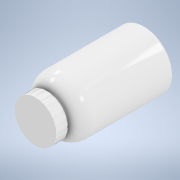
# Autodesk Inventor part: Healing-Iteam-Pills
Saved by Autodesk Inventor 2020 (Build 240168000, 168)
## iProperties
Created: 2019-09-13
Part Number: Healing-Iteam-Pills
Material: Generic
Document SubType Name: Modeling
Designer: vifly_01
Density: 1 g/cm^3
Appearance: Default
Author: vifly_01
Autodesk Inventor part; units mm, degrees
ref_plane "YZ Plane" through (0, 0, 0) normal (1, 0, 0) x (0, 1, 0)
ref_plane "XZ Plane" through (0, 0, 0) normal (0, 1, 0) x (-1, 0, 0)
ref_plane "XY Plane" through (0, 0, 0) normal (0, 0, 1) x (1, 0, 0)
sketch "Sketch1" plane through (0, 0, 0) normal (0, 0, 1) x (1, 0, 0)
  circle A0 centre (0, 0) radius 7.5
  dimension "d0" = 15
  constraints: 1 centre point, 1 coincident
  measures "d0" diameter of A0
extrude "Extrusion1" add sketch "Sketch1" along normal blind 20
sketch "Sketch3" plane through (0, 0, 0) normal (1, 0, 0) x (0, 1, 0)
  line L0 (7.5, 20) -> (-7.5, 20) projected
  arc A0 (7.5, 20) -> (4.75, 25) centre (2.4104, 20.457) ccw
  line L1 (4.75, 25) -> (4.75, 20)
  line L2 (7.5, 20) -> (4.75, 20)
  line L3 (0, -5.128) -> (0, 30.7682) projected
  point P0 (0, 0)
  dimension "d3" = 5
  dimension "d4" = 2.75
  constraints: 4 end point, 2 point on circle, 1 centre point, 1 collinear, 1 perpendicular, 1 point on line
  measures "d3" distance from line of L0 L1.start
  measures "d4" horizontal distance of L0.start L1.start
revolve "Revolution1" add sketch "Sketch3" angle 360 about axis through (0, 0, -10) along (0, 0, 1)
sketch "Sketch4" plane through (0, 0, 20) normal (0, 0, 1) x (1, 0, 0)
  circle A0 centre (0, 0) radius 4.75
  constraints: 1 centre point, 1 coincident
extrude "Extrusion2" add sketch "Sketch4" along normal blind 5.75
sketch "Sketch5" plane through (0, 0, 25.75) normal (0, 0, 1) x (1, 0, 0)
  circle A0 centre (0, 0) radius 5.5
  dimension "d8" = 11
  constraints: 1 centre point, 1 coincident
  measures "d8" diameter of A0
extrude "Extrusion3" add sketch "Sketch5" along normal blind 3
sketch "Sketch6" plane through (0, 0, 28.75) normal (0, 0, 1) x (1, 0, 0)
  arc A0 (-5.4899, 0.3337) -> (-5.5, 0) centre (0, 0) ccw
  circle A1 centre (0, 0) radius 5.5 projected
  arc A2 (-5.4398, 0.3337) -> (-5.45, 0) centre (0, 0) ccw
  line L0 (-5.4398, 0.3337) -> (-5.4899, 0.3337)
  line L1 (-5.45, 0) -> (-5.5, 0)
  line L2 (-5.6591, 0) -> (-5.2331, 0)
  arc A3 (-5.5, 0) -> (-5.4899, -0.3337) centre (0, 0) ccw
  arc A4 (-5.45, 0) -> (-5.4398, -0.3337) centre (0, 0) ccw
  line L3 (-5.4398, -0.3337) -> (-5.4899, -0.3337)
  point P0 (-5.4899, -0.3337)
  dimension "d14" = 0.05
  constraints: 10 point on circle, 8 end point, 4 centre point, 2 horizontal, 2 symmetric about line, 1 coincident, 1 parallel, 2 other
  measures "d14" radial gap between concentric circles of A0 A2
extrude "Extrusion4" cut sketch "Sketch6" against normal blind 3 contours L0 A2 L1 A0 | L1 A4 L3 A1
pattern_circular "Circular Pattern1" count 20 over 360 about axis through (0, 0, 25.75) along (0, 0, 1) of "Extrusion4"
fillet "Fillet1" radius 0.5 1 edges at (-7.5, 0, 0)
body "Solid1"
